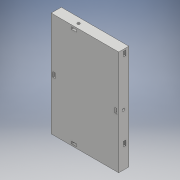
# Autodesk Inventor part: Case_Top
Saved by Autodesk Inventor 2019 (Build 230136000, 136)
## iProperties
Created: 2019-02-05
Part Number: Case_Top
Material: Generic
Document SubType Name: Modeling
Designer: Jorian Bruslind
Density: 1 g/cm^3
Appearance: Default
Author: Jorian Bruslind
Autodesk Inventor part; units mm, degrees
ref_plane "YZ Plane" through (0, 0, 0) normal (1, 0, 0) x (0, 1, 0)
ref_plane "XZ Plane" through (0, 0, 0) normal (0, 1, 0) x (-1, 0, 0)
ref_plane "XY Plane" through (0, 0, 0) normal (0, 0, 1) x (1, 0, 0)
sketch "Sketch1" plane through (0, 0, 0) normal (0, 1, 0) x (-1, 0, 0)
  line L0 (0, 0) -> (80, 0)
  line L1 (80, 0) -> (80, -124)
  line L2 (80, -124) -> (0, -124)
  line L3 (0, -124) -> (0, 0)
  dimension "d0" = 80
  dimension "d1" = 124
  constraints: 8 end point, 2 parallel, 1 horizontal, 1 perpendicular
  measures "d0" distance of L1.end L2.end
  measures "d1" distance of L0.end L1.end
extrude "Extrusion1" add sketch "Sketch1" along normal blind 12
sketch "Sketch2" plane through (0, 12, 0) normal (0, 1, 0) x (1, 0, 0)
  line L0 (0, 0) -> (0, 124) projected
  line L1 (0, 124) -> (-2, 124)
  line L2 (0, 124) -> (-80, 124) projected
  line L3 (-2, 124) -> (-2, 122)
  line L4 (-2, 122) -> (-78, 122)
  line L5 (-78, 122) -> (-78, 2)
  line L6 (-78, 2) -> (-2, 2)
  line L7 (-2, 2) -> (-2, 122)
  dimension "d4" = 2
  dimension "d5" = 2
  dimension "d6" = 270
  dimension "d7" = 76
  dimension "d8" = 120
  constraints: 12 end point, 2 parallel, 2 perpendicular, 1 horizontal, 1 point on line
  measures "d4" distance of L0.end L1.end
  measures "d5" distance of L1.end L3.end
  measures "d7" distance of L5.end L6.end
  measures "d8" distance of L4.end L5.end
extrude "Extrusion2" cut sketch "Sketch2" against normal blind 10
sketch "Sketch5" plane through (0, 2, 0) normal (0, 1, 0) x (1, 0, 0)
  line L0 (-2, 2) -> (-78, 2) projected
  line L1 (-2, 2) -> (-10, 2)
  line L2 (-10, 2) -> (-10, 10)
  line L3 (-10, 10) -> (-2, 10)
  line L4 (-2, 10) -> (-2, 2)
  line L5 (-2, 2) -> (-4.5, 2)
  line L6 (-4.5, 2) -> (-4.5, 5)
  line L7 (-78, 2) -> (-70, 2)
  line L8 (-70, 2) -> (-70, 10)
  line L9 (-70, 10) -> (-78, 10)
  line L10 (-78, 10) -> (-78, 2)
  line L11 (-2, 2) -> (-78, 2) projected
  line L12 (-78, 2) -> (-78, 101.45)
  line L13 (-78, 2) -> (21.45, 2) construction
  line L14 (-2, 122) -> (-2, 2) projected
  line L15 (-2, 2) -> (-2, 101.45)
  line L16 (-2, 2) -> (97.45, 2) construction
  line L17 (-78, 101.45) -> (-70, 101.45)
  line L18 (-70, 101.45) -> (-70, 93.45)
  line L19 (-70, 93.45) -> (-78, 93.45)
  line L20 (-78, 93.45) -> (-78, 101.45)
  line L21 (-2, 101.45) -> (-10, 101.45)
  line L22 (-10, 101.45) -> (-10, 93.45)
  line L23 (-10, 93.45) -> (-2, 93.45)
  line L24 (-2, 93.45) -> (-2, 101.45)
  point P0 (0, 0)
  dimension "d31" = 8
  dimension "d32" = 8
  dimension "d34" = 2.5
  dimension "d35" = 3
  dimension "d36" = 8
  dimension "d37" = 8
  dimension "d83" = 99.45
  dimension "d84" = 90
  dimension "d85" = 99.45
  dimension "d86" = 90
  dimension "d87" = 8
  dimension "d88" = 8
  dimension "d89" = 8
  dimension "d90" = 8
  constraints: 44 end point, 8 parallel, 8 perpendicular, 6 horizontal, 1 collinear, 1 point on line
  measures "d31" distance of L2.end L3.end
  measures "d32" distance of L1.end L2.end
  measures "d34" distance of L0.start L5.end
  measures "d35" distance of L5.end L6.end
  measures "d36" distance of L9.end L8.end
  measures "d37" distance of L8.end L7.end
  measures "d83" distance of L0.end L12.end
  measures "d84" angle of L13 L12
  measures "d85" distance of L0.start L15.end
  measures "d86" angle of L16 L15
  measures "d87" distance of L18.end L19.end
  measures "d88" distance of L17.end L18.end
  measures "d89" distance of L23.end L22.end
  measures "d90" distance of L22.end L21.end
extrude "Extrusion8" add sketch "Sketch5" along normal blind 10
sketch "Sketch9" plane through (0, 12, 0) normal (0, 1, 0) x (1, 0, 0)
  circle A0 centre (-5.5701, 5) radius 1.5
  circle A1 centre (-75.5, 5) radius 1.5
  circle A2 centre (-4.5, 97.45) radius 1.5
  circle A3 centre (-75.5, 97.45) radius 1.5
  line L0 (-70, 101.45) -> (-78, 101.45) projected
  line L1 (-78, 10) -> (-78, 93.45) projected
  line L2 (-10, 2) -> (-70, 2) projected
  line L3 (-10, 10) -> (-10, 2) projected
  line L4 (-10, 93.45) -> (-2, 93.45) projected
  line L5 (-2, 93.45) -> (-2, 10) projected
  point P0 (0, 0)
  dimension "d93" = 4
  dimension "d94" = 2.5
  dimension "d95" = 3
  dimension "d96" = 2.5
  dimension "d97" = 3
  dimension "d98" = 4.4299
  dimension "d99" = 3
  dimension "d100" = 4
  dimension "d101" = 2.5
  constraints: 4 centre point, 3 equal radius
  measures "d93" distance from line of L0 A3.centre
  measures "d94" distance from line of L1 A3.centre
  measures "d95" diameter of A3
  measures "d96" distance from line of L1 A1.centre
  measures "d97" distance from line of L2 A1.centre
  measures "d98" distance from line of L3 A0.centre
  measures "d99" distance from line of L2 A0.centre
  measures "d100" distance from line of L4 A2.centre
  measures "d101" distance from line of L5 A2.centre
extrude "Extrusion9" cut sketch "Sketch9" against normal blind 10
sketch "Sketch11" plane through (0, 0, -124) normal (0, 0, -1) x (-1, 0, 0)
  line L0 (80, 0) -> (80, 12) projected
  line L1 (80, 0) -> (53, 0)
  line L2 (0, 0) -> (80, 0) projected
  line L3 (53, 0) -> (53, 5.5)
  circle A0 centre (53, 5.5) radius 1.5
  dimension "d107" = 27
  dimension "d108" = 5.5
  dimension "d109" = 3
  constraints: 4 end point, 1 centre point, 1 coincident, 1 perpendicular, 1 point on line
  measures "d107" distance of L0.start L1.end
  measures "d108" distance of L1.end L3.end
  measures "d109" diameter of A0
sketch "Sketch12" plane through (0, 0, 0) normal (1, 0, 0) x (0, 0, -1)
  line L0 (0, 0) -> (0, 12) projected
  line L1 (0, 0) -> (0, 5.85)
  line L2 (0, 5.85) -> (2.125, 5.85)
  line L3 (2.125, 5.85) -> (7.875, 5.85)
  line L4 (7.875, 5.85) -> (7.875, 8.45)
  line L5 (7.875, 8.45) -> (2.125, 8.45)
  line L6 (2.125, 8.45) -> (2.125, 5.85)
  line L7 (124, 0) -> (0, 0) projected
  line L8 (7.875, 5.85) -> (94.575, 5.85)
  line L9 (10, 12) -> (10, 2) projected
  line L10 (7.875, 5.85) -> (94.575, 5.85) construction
  line L11 (94.575, 5.85) -> (100.325, 5.85)
  line L12 (100.325, 5.85) -> (100.325, 8.45)
  line L13 (100.325, 8.45) -> (94.575, 8.45)
  line L14 (94.575, 8.45) -> (94.575, 5.85)
  dimension "d112" = 5.85
  dimension "d113" = 2.125
  dimension "d114" = 5.75
  dimension "d115" = 2.6
  dimension "d122" = 86.7
  dimension "d123" = 0
  dimension "d124" = 5.75
  dimension "d125" = 2.6
  constraints: 24 end point, 4 parallel, 4 perpendicular, 3 horizontal, 1 collinear, 1 point on line
  measures "d112" distance of L0.start L1.end
  measures "d113" distance of L1.end L2.end
  measures "d114" distance of L5.end L4.end
  measures "d115" distance of L4.end L3.end
  measures "d122" distance of L3.end L8.end
  measures "d123" distance between parallel lines of L8 L10
  measures "d124" distance of L13.end L12.end
  measures "d125" distance of L12.end L11.end
extrude "Extrusion11" cut sketch "Sketch12" against normal blind 8
sketch "Sketch13" plane through (-80, 0, -124) normal (-1, 0, 0) x (0, 0, 1)
  line L0 (124, 0) -> (124, 5.85)
  line L1 (124, 0) -> (124, 12) projected
  line L2 (124, 5.85) -> (121.875, 5.85)
  line L3 (121.875, 5.85) -> (116.125, 5.85)
  line L4 (116.125, 5.85) -> (116.125, 8.45)
  line L5 (116.125, 8.45) -> (121.875, 8.45)
  line L6 (121.875, 8.45) -> (121.875, 5.85)
  line L7 (116.125, 5.85) -> (29.425, 5.85)
  line L8 (114, 2) -> (114, 12) projected
  line L9 (116.125, 5.85) -> (202.825, 5.85) construction
  line L10 (29.425, 5.85) -> (23.675, 5.85)
  line L11 (23.675, 5.85) -> (23.675, 8.45)
  line L12 (23.675, 8.45) -> (29.425, 8.45)
  line L13 (29.425, 8.45) -> (29.425, 5.85)
  dimension "d126" = 5.85
  dimension "d127" = 2.125
  dimension "d128" = 5.75
  dimension "d129" = 2.6
  dimension "d130" = 86.7
  dimension "d131" = 180
  dimension "d132" = 5.75
  dimension "d181" = 2.6
  constraints: 24 end point, 4 parallel, 4 perpendicular, 3 horizontal, 1 collinear, 1 point on line
  measures "d126" distance of L0.start L0.end
  measures "d127" distance of L0.end L2.end
  measures "d128" distance of L4.end L5.end
  measures "d129" distance of L3.end L4.end
  measures "d130" distance of L3.end L7.end
  measures "d131" angle of L7 L9
  measures "d132" distance of L11.end L12.end
  measures "d181" distance of L12.end L7.end
extrude "Extrusion12" cut sketch "Sketch13" against normal blind 8
sketch "Sketch14" plane through (0, 0, 0) normal (1, 0, 0) x (0, 0, -1)
  line L0 (0, 0) -> (124, 0) projected
  line L1 (0, 0) -> (62, 0)
  line L2 (62, 0) -> (62, 5.5)
  circle A0 centre (62, 5.5) radius 1.5
  line L3 (0, 0) -> (0, 12) projected
  dimension "d135" = 5.5
  dimension "d136" = 3
  dimension "d139" = 62
  constraints: 4 end point, 1 centre point, 1 coincident, 1 midpoint, 1 vertical
  measures "d135" distance of L1.end L2.end
  measures "d136" diameter of A0
  measures "d139" distance from line of L3 L2.end
sketch "Sketch15" plane through (0, 2, 0) normal (0, 1, 0) x (1, 0, 0)
  line L0 (-80, 0) -> (0, 0) projected
  line L1 (-80, 0) -> (-56.75, 0)
  line L2 (-56.75, 0) -> (-56.75, 2)
  line L3 (-10, 2) -> (-70, 2) projected
  line L4 (-56.75, 2) -> (-49.25, 2)
  line L5 (-49.25, 2) -> (-49.25, 6)
  line L6 (-49.25, 6) -> (-56.75, 6)
  line L7 (-56.75, 6) -> (-56.75, 2)
  line L8 (0, 124) -> (-80, 124) projected
  line L9 (-80, 124) -> (-56.75, 124)
  line L10 (-56.75, 124) -> (-56.75, 122)
  line L11 (-78, 122) -> (-2, 122) projected
  line L12 (-56.75, 122) -> (-49.25, 122)
  line L13 (-49.25, 122) -> (-49.25, 118)
  line L14 (-49.25, 118) -> (-56.75, 118)
  line L15 (-56.75, 118) -> (-56.75, 122)
  line L16 (0, 0) -> (0, 58.75)
  line L17 (0, 0) -> (0, 124) projected
  line L18 (0, 58.75) -> (-2, 58.75)
  line L19 (-2, 93.45) -> (-2, 10) projected
  line L20 (-2, 58.75) -> (-6, 58.75)
  line L21 (-6, 58.75) -> (-6, 66.25)
  line L22 (-6, 66.25) -> (-2, 66.25)
  line L23 (-2, 66.25) -> (-2, 58.75)
  line L24 (-80, 0) -> (-80, 58.75)
  line L25 (-80, 124) -> (-80, 0) projected
  line L26 (-80, 58.75) -> (-78, 58.75)
  line L27 (-78, 10) -> (-78, 93.45) projected
  line L28 (-78, 58.75) -> (-74, 58.75)
  line L29 (-74, 58.75) -> (-74, 66.25)
  line L30 (-74, 66.25) -> (-78, 66.25)
  line L31 (-78, 66.25) -> (-78, 58.75)
  dimension "d140" = 23.25
  dimension "d141" = 7.5
  dimension "d142" = 4
  dimension "d143" = 23.25
  dimension "d144" = 7.5
  dimension "d145" = 4
  dimension "d146" = 58.75
  dimension "d147" = 4
  dimension "d148" = 7.5
  dimension "d149" = 58.75
  dimension "d150" = 4
  dimension "d151" = 7.5
  constraints: 48 end point, 8 parallel, 8 point on line, 6 perpendicular, 4 horizontal, 2 vertical
  measures "d140" distance of L0.start L1.end
  measures "d141" distance of L6.end L5.end
  measures "d142" distance of L5.end L4.end
  measures "d143" distance of L8.end L9.end
  measures "d144" distance of L13.end L14.end
  measures "d145" distance of L12.end L13.end
  measures "d146" distance of L0.end L16.end
  measures "d147" distance of L21.end L22.end
  measures "d148" distance of L20.end L21.end
  measures "d149" distance of L0.start L24.end
  measures "d150" distance of L30.end L29.end
  measures "d151" distance of L29.end L28.end
extrude "Extrusion14" add sketch "Sketch15" along normal blind 10 contours L7 L6 L5 L3 | L20 L21 L22 L19 | L11 L13 L14 L15 | L27 L30 L29 L28
extrude "Extrusion15" cut sketch "Sketch11" against normal blind 124
extrude "Extrusion16" cut sketch "Sketch14" against normal blind 82
sketch "Sketch16" plane through (0, 0, 0) normal (0, -1, 0) x (1, 0, 0)
  line L0 (-80, 0) -> (0, 0) projected
  line L1 (-80, 0) -> (-55.875, 0)
  line L2 (-55.875, 0) -> (-55.875, -2)
  line L3 (-55.875, -2) -> (-50.125, -2)
  line L4 (-50.125, -2) -> (-50.125, -4.6)
  line L5 (-50.125, -4.6) -> (-55.875, -4.6)
  line L6 (-55.875, -4.6) -> (-55.875, -2)
  line L7 (0, -124) -> (-80, -124) projected
  line L8 (-80, -124) -> (-55.875, -124)
  line L9 (-55.875, -124) -> (-55.875, -122)
  line L10 (-55.875, -122) -> (-50.125, -122)
  line L11 (-50.125, -122) -> (-50.125, -119.4)
  line L12 (-50.125, -119.4) -> (-55.875, -119.4)
  line L13 (-55.875, -119.4) -> (-55.875, -122)
  line L14 (-80, 0) -> (-80, -59.125)
  line L15 (-80, 0) -> (-80, -124) projected
  line L16 (-80, 0) -> (-20.875, 0) construction
  line L17 (-80, -59.125) -> (-78, -59.125)
  line L18 (-74, -60.5) -> (-74, -63.5) projected
  line L19 (-78, -59.125) -> (-75.4, -59.125)
  line L20 (-75.4, -59.125) -> (-75.4, -64.875)
  line L21 (-75.4, -64.875) -> (-78, -64.875)
  line L22 (-78, -64.875) -> (-78, -59.125)
  line L23 (0, 0) -> (0, -59.125)
  line L24 (-2, -58.75) -> (-2, -10) projected
  line L25 (0, 0) -> (59.125, 0) construction
  line L26 (0, -59.125) -> (-2, -59.125)
  line L27 (0, -63.5) -> (-6, -63.5) projected
  line L28 (-2, -59.125) -> (-4.6, -59.125)
  line L29 (-4.6, -59.125) -> (-4.6, -64.875)
  line L30 (-4.6, -64.875) -> (-2, -64.875)
  line L31 (-2, -64.875) -> (-2, -59.125)
  dimension "d158" = 24.125
  dimension "d162" = 2
  dimension "d163" = 5.75
  dimension "d164" = 2.6
  dimension "d165" = 24.125
  dimension "d166" = 2
  dimension "d167" = 5.75
  dimension "d168" = 2.6
  dimension "d169" = 59.125
  dimension "d170" = 90
  dimension "d171" = 2
  dimension "d172" = 2.6
  dimension "d173" = 5.75
  dimension "d174" = 59.125
  dimension "d175" = 90
  dimension "d176" = 2
  dimension "d177" = 2.6
  dimension "d178" = 5.75
  constraints: 52 end point, 10 parallel, 8 perpendicular, 6 horizontal, 2 point on line, 1 collinear, 1 vertical
  measures "d158" distance of L0.start L1.end
  measures "d162" distance of L1.end L2.end
  measures "d163" distance of L4.end L5.end
  measures "d164" distance of L3.end L4.end
  measures "d165" distance of L7.end L8.end
  measures "d166" distance of L8.end L9.end
  measures "d167" distance of L12.end L11.end
  measures "d168" distance of L11.end L10.end
  measures "d169" distance of L0.start L14.end
  measures "d170" angle of L14 L16
  measures "d171" distance of L14.end L17.end
  measures "d172" distance of L20.end L21.end
  measures "d173" distance of L19.end L20.end
  measures "d174" distance of L0.end L23.end
  measures "d175" angle of L23 L25
  measures "d176" distance of L23.end L26.end
  measures "d177" distance of L30.end L29.end
  measures "d178" distance of L29.end L28.end
extrude "Extrusion17" cut sketch "Sketch16" against normal blind 8.5
body "Solid1"
